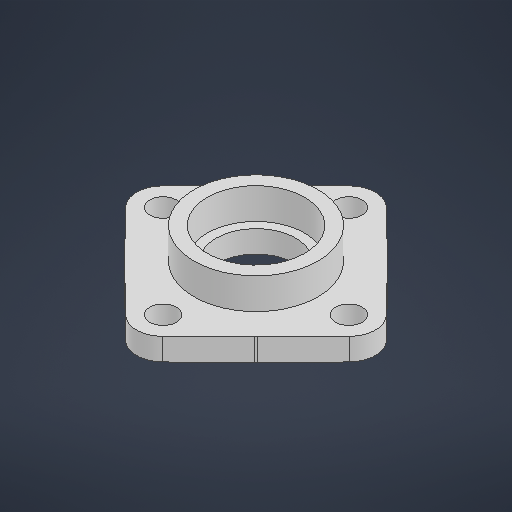
# Autodesk Inventor part: rodamiento_shell
Saved by Autodesk Inventor 2025 (Build 290162010, 162A)
## iProperties
Created: 2024-11-09
Part Number: rodamiento_shell
Material: Generic
Document SubType Name: Modeling
Designer: river
Density: 1 g/cm^3
Appearance: Default
Author: river
Autodesk Inventor part; units mm, degrees
ref_plane "YZ Plane" through (0, 0, 0) normal (1, 0, 0) x (0, 1, 0)
ref_plane "XZ Plane" through (0, 0, 0) normal (0, 1, 0) x (-1, 0, 0)
ref_plane "XY Plane" through (0, 0, 0) normal (0, 0, 1) x (1, 0, 0)
derived "lamina_estator.ipt"
sketch "Sketch3" plane through (0, 3, 0) normal (0, 1, 0) x (1, 0, 0)
  circle A0 centre (-21, 0) radius 3 projected
  line L0 (0, 0) -> (-21, 0) construction
  circle A1 centre (0, -21) radius 3 projected
  circle A2 centre (21, 0) radius 3 projected
  circle A3 centre (0, 0) radius 14 projected
  circle A4 centre (0, 21) radius 3 projected
  circle A5 centre (0, 0) radius 11
  circle A6 centre (-21, 0) radius 6
  circle A7 centre (0, -21) radius 6
  circle A8 centre (21, 0) radius 6
  circle A9 centre (0, 21) radius 6
  circle A10 centre (0, 0) radius 9
  circle A11 centre (0, 0) radius 21
  line L1 (-14.6969, 15) -> (-4.1991, 25.2857)
  line L2 (4.1991, 25.2857) -> (14.6969, 15)
  line L3 (-15, -14.6969) -> (-25.2857, -4.1991)
  line L4 (-25.2857, 4.1991) -> (-15, 14.6969)
  line L5 (14.6969, -15) -> (4.1991, -25.2857)
  line L6 (-4.1991, -25.2857) -> (-14.6969, -15)
  line L7 (15, 14.6969) -> (25.2857, 4.1991)
  line L8 (25.2857, -4.1991) -> (15, -14.6969)
  point P0 (25.2857, 4.1991)
  dimension "d1" = 22
  dimension "d2" = 12
  dimension "d5" = 360
  dimension "d15" = 18
  dimension "d21" = 360
  constraints: 16 end point, 7 centre point, 5 point on circle, 4 coincident, 4 tangent, 35 other
  measures "d1" diameter of A5
  measures "d2" diameter of A6
  measures "d15" diameter of A10
extrude "Extrusion4" add sketch "Sketch3" along normal blind 7 contours A3
extrude "Extrusion5" add sketch "Sketch3" against normal blind 5 contours A0 A11 A6 | A0 A11 A6 | A11 A9 A8 A7 A6 | A6 L4 A11 | A11 L3 A6 | L1 A9 A11 | A11 A7 L6 | A11 A4 A9 | A9 A11 A4 | A11 A1 A7 | A7 A11 A1 | A9 L2 A11 | A11 L5 A7 | L7 A8 A11 | A11 A8 L8 | A11 A2 A8 | A8 A11 A2 | A3 | A5
body "Solid3"
